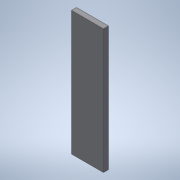
# Autodesk Inventor part: LeftBoxCover
Saved by Autodesk Inventor 2020 (Build 240168000, 168)
## iProperties
Created: 2019-06-03
Part Number: LeftBoxCover
Material: Generic
Document SubType Name: Modeling
Designer: LillaHunden
Density: 1 g/cm^3
Appearance: Default
Author: LillaHunden
Autodesk Inventor part; units mm, degrees
ref_plane "YZ Plane" through (0, 0, 0) normal (1, 0, 0) x (0, 1, 0)
ref_plane "XZ Plane" through (0, 0, 0) normal (0, 1, 0) x (-1, 0, 0)
ref_plane "XY Plane" through (0, 0, 0) normal (0, 0, 1) x (1, 0, 0)
sketch "Sketch1" plane through (0, 0, 0) normal (0, 0, 1) x (1, 0, 0)
  line L0 (67, 4) -> (76.9823, 4) construction
  line L1 (76.9823, 4) -> (76.9823, 12) construction
  line L2 (0, 12) -> (76.9823, 12) construction
  line L3 (0, 0) -> (0, 12) construction
  line L4 (67, 0) -> (0, 0) construction
  line L5 (67, 0) -> (67, 4) construction
  line L6 (67, -280) -> (67, -276) construction
  line L7 (67, -276) -> (0, -276) construction
  line L8 (0, -276) -> (0, -288) construction
  line L9 (76.9823, -288) -> (0, -288) construction
  line L10 (76.9823, -280) -> (76.9823, -288) construction
  line L11 (76.9823, -280) -> (67, -280) construction
  line L12 (76.9823, 12) -> (0, 12)
  line L13 (0, 12) -> (0, -288)
  line L14 (0, -288) -> (76.9823, -288)
  line L15 (76.9823, -288) -> (76.9823, 12)
  constraints: 8 end point, 2 parallel, 1 horizontal, 1 perpendicular
extrude "Extrusion1" add sketch "Sketch1" along normal blind 12
sketch "Sketch2" plane through (0, 0, 0) normal (0, 0, -1) x (-1, 0, 0)
  line L0 (-76.9823, -280) -> (-67, -280) construction
  line L1 (-67, -276) -> (0, -276) construction
  line L2 (-67, -280) -> (-67, -276) construction
  line L3 (0, -275.9) -> (-67.1, -275.9)
  line L4 (-67.1, -275.9) -> (-67.1, -279.9)
  line L5 (-67.1, -279.9) -> (-76.9823, -279.9)
  line L6 (0, 12) -> (0, -288) projected
  line L7 (-76.9823, 12) -> (0, 12) projected
  line L8 (-76.9823, -288) -> (-76.9823, 12) projected
  line L9 (0, -288) -> (-76.9823, -288) projected
  point P0 (0, 0)
  dimension "d2" = 0.1
  constraints: 6 end point, 2 other
  measures "d2" distance between parallel lines of L1 L3
extrude "Extrusion2" cut sketch "Sketch2" against normal blind 8.75 contours L6 L9 L8 L5 L4 L3
sketch "Sketch3" plane through (0, 0, 0) normal (0, 0, -1) x (-1, 0, 0)
  line L0 (-67, 4) -> (-76.9823, 4) construction
  line L1 (-67, 0) -> (0, 0) construction
  line L2 (-67, 0) -> (-67, 4) construction
  line L3 (-76.9823, 3.9) -> (-67.1, 3.9)
  line L4 (-67.1, 3.9) -> (-67.1, -0.1)
  line L5 (-67.1, -0.1) -> (0, -0.1)
  line L6 (-67.1, -275.9) -> (0, -275.9) projected
  line L7 (0, 12) -> (0, -275.9) projected
  line L8 (-76.9823, 12) -> (0, 12) projected
  line L9 (-76.9823, -279.9) -> (-76.9823, 12) projected
  line L10 (-76.9823, -279.9) -> (-67.1, -279.9) projected
  line L11 (-67.1, -279.9) -> (-67.1, -275.9) projected
  point P0 (0, -0.1)
  dimension "d5" = 0.1
  constraints: 6 end point, 2 other
  measures "d5" distance between parallel lines of L0 L3
extrude "Extrusion3" cut sketch "Sketch3" against normal up to surface (8.75 mm away) contours L9 L8 L7 L5 L4 L3
sketch "Sketch4" plane through (76.9823, -288, 12) normal (1, 0, 0) x (0, 0, -1)
  line L0 (3.25, 291.9) -> (3.25, 300) projected
  line L1 (12, 8.1) -> (12, 291.9) projected
  line L2 (3.25, 291.9) -> (12, 291.9)
  line L3 (12, 291.9) -> (12, 161.7)
  line L4 (12, 161.7) -> (3.25, 161.7)
  line L5 (3.25, 161.7) -> (3.25, 291.9)
  line L6 (196.25, 162) -> (3.25, 162) construction
  point P0 (12, 288)
  dimension "d8" = 0.3
  constraints: 8 end point, 2 parallel, 1 horizontal, 1 perpendicular, 1 point on line
  measures "d8" distance between parallel lines of L6 L4
ref_plane "Work Plane1" through (48, -120, -184.25) normal (-1, 0, 0) x (0, 0, 1)
extrude "Extrusion4" cut sketch "Sketch4" against normal up to surface (28.9823 mm away) draft 0.3
sketch "Sketch5" plane through (48, -126.4518, 8.9018) normal (1, 0, 0) x (0, 0, -1)
  arc A0 (6.828, 119.8758) -> (6.828, 114.6758) centre (6.828, 117.2758) ccw construction
  line L0 (6.828, 119.8758) -> (21.628, 119.8758) construction
  line L1 (21.628, 114.6758) -> (6.828, 114.6758) construction
  arc A1 (6.828, 72.7358) -> (6.828, 67.5358) centre (6.828, 70.1358) ccw construction
  line L2 (21.628, 67.5358) -> (6.828, 67.5358) construction
  line L3 (6.828, 72.7358) -> (21.628, 72.7358) construction
  line L4 (21.628, 113.1758) -> (6.828, 113.1758)
  arc A2 (6.828, 121.3758) -> (6.828, 113.1758) centre (6.828, 117.2758) ccw
  line L5 (6.828, 121.3758) -> (21.628, 121.3758)
  line L6 (21.628, 66.0358) -> (6.828, 66.0358)
  arc A3 (6.828, 74.2358) -> (6.828, 66.0358) centre (6.828, 70.1358) ccw
  line L7 (6.828, 74.2358) -> (21.628, 74.2358)
  line L8 (8.9018, 126.3518) -> (8.9018, 0) projected
  line L9 (8.9018, 113.1758) -> (8.9018, 121.3758)
  line L10 (8.9018, 74.2358) -> (8.9018, 66.0358)
  point P0 (8.9018, 126.4518)
  point P1 (8.9018, 74.2358)
  dimension "d11" = 1.5
  dimension "d12" = 1.5
  constraints: 12 end point, 8 point on line, 4 point on circle, 2 centre point, 4 other
  measures "d11" radial gap between concentric circles of A0 A2
  measures "d12" radial gap between concentric circles of A1 A3
extrude "Extrusion5" cut sketch "Sketch5" against normal blind 6
sketch "Sketch6" plane through (48, -126.4518, 8.9018) normal (1, 0, 0) x (0, 0, -1)
  line L0 (193.1518, 6.4518) -> (0.1518, 6.4518) construction
  line L1 (0.1518, 6.4518) -> (0.1518, 0.4518) construction
  line L2 (193.1518, 0.4518) -> (0.1518, 0.4518) construction
  line L3 (193.1518, 6.4518) -> (193.1518, 0.4518) construction
  line L4 (0.1518, 10.4518) -> (193.1518, 10.4518) construction
  line L5 (0.1518, 0.4518) -> (193.1518, 0.4518) construction
  line L6 (0.1518, 0.1518) -> (0, 0) projected
  line L7 (8.9018, 66.0358) -> (8.9018, 0) projected
  line L8 (0, 0) -> (8.9018, 0)
  line L9 (8.9018, 0) -> (8.9018, 10.7518)
  line L10 (8.9018, 10.7518) -> (0, 10.7518)
  line L11 (0, 10.7518) -> (0, 0)
  point P0 (8.9018, 126.4518)
  dimension "d15" = 0.3
  constraints: 8 end point, 2 parallel, 1 horizontal, 1 perpendicular, 1 point on line
  measures "d15" distance between parallel lines of L10 L4
extrude "Extrusion6" cut sketch "Sketch6" against normal through all
body "Solid1"
